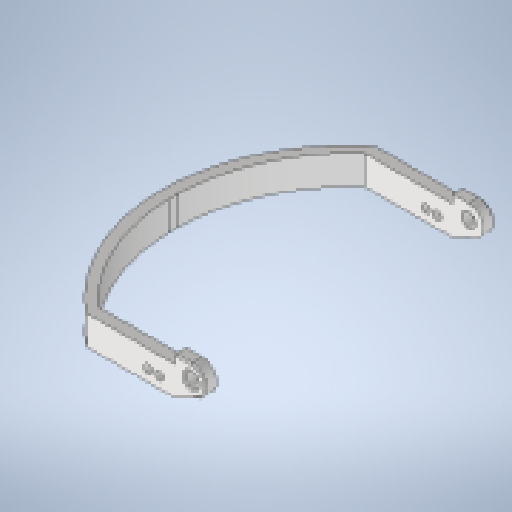
# Autodesk Inventor part: Gripper_v1
Saved by Autodesk Inventor 2025.1 (Build 291241000, 241)
## iProperties
Created: 2026-05-06
Part Number: Gripper_v1
Material: Generic
Document SubType Name: Modeling
Designer: User
Density: 1 g/cm^3
Appearance: Default
Author: User
## iProperties of the stored document Gripper_v1_3DPrint.ipt
Created: 2026-05-06
Part Number: Gripper_v1_3DPrint
Material: Generic
Document SubType Name: Modeling
Designer: User
Density: 1 g/cm^3
Appearance: Default
Author: User
Autodesk Inventor part; units mm, degrees
ref_plane "YZ Plane" through (0, 0, 0) normal (1, 0, 0) x (0, 1, 0)
ref_plane "XZ Plane" through (0, 0, 0) normal (0, 1, 0) x (-1, 0, 0)
ref_plane "XY Plane" through (0, 0, 0) normal (0, 0, 1) x (1, 0, 0)
sketch "Sketch1" plane through (0, 0, 0) normal (0, 0, 1) x (1, 0, 0)
  circle A0 centre (0, 0) radius 2.5 projected
  circle A1 centre (0, 0) radius 2.6
  circle A2 centre (0, 0) radius 5.1
  point P0 (0, 0)
  dimension "d0" = 0.1
  dimension "d1" = 2.5
  constraints: 2 centre point
  measures "d0" radial gap between concentric circles of A0 A1
  measures "d1" radial gap between concentric circles of A1 A2
ref_plane "Work Plane1" through (-3.6464, -27.211, -4) normal (0, 0, 1) x (1, 0, 0)
extrude "Extrusion1" add sketch "Sketch1" against normal up to surface (4 mm away) contours A2
chamfer "Chamfer1" distance 0.5 angle 45 1 edges at (-2.6, 0, -4)
sketch "Sketch2" plane through (0, 0, 0) normal (0, 0, 1) x (1, 0, 0)
  circle A0 centre (0, 0) radius 5.1 projected
  line L0 (-5.6464, 6) -> (-5.6464, -27.211) projected
  circle A1 centre (0, 0) radius 5.1 projected
  line L1 (0, -5.1) -> (-5.6464, -5.1)
  line L2 (0, 5.1) -> (-5.6464, 5.1)
  point P0 (0, 0)
  constraints: 4 end point, 3 tangent, 2 perpendicular, 2 point on circle, 2 point on line
extrude "Extrusion2" add sketch "Sketch2" against normal up to surface (4 mm away) contours A0 L1 L0 L2
sketch "Sketch5" plane through (-5.6464, -5.1, 0) normal (-1, 0, 0) x (0, 0, 1)
  line L0 (-4, 0) -> (-4, 10.2) projected
  line L1 (0, 0) -> (-4, 0) projected
  line L2 (0, 10.2) -> (0, 0) projected
  line L3 (0, 10.2) -> (-4, 10.2) projected
  line L4 (0, 0) -> (0, -3)
  line L5 (0, -3) -> (-4, -3)
  line L6 (-4, 10.2) -> (-4, 7.2)
  line L7 (-4, 7.2) -> (0, 7.2)
  line L8 (0, 7.2) -> (0, -3)
  line L9 (0, -3) -> (-4, -3)
  line L10 (-4, -3) -> (-4, 7.2)
  point P0 (0, 5.1)
  dimension "d14" = 3
  dimension "d15" = 3
  constraints: 14 end point, 2 parallel, 2 perpendicular, 1 horizontal, 1 point on line, 1 vertical
  measures "d14" distance of L1.start L4.end
  measures "d15" distance of L0.end L6.end
extrude "Extrusion5" add sketch "Sketch5" along normal blind 1 contours L0 L7 L2 L1 | L1 L4 L5 L10
sketch "Sketch6" plane through (0, 0, 0) normal (0, 0, 1) x (1, 0, 0)
  line L0 (-5.6464, -5.1) -> (0, -5.1) projected
  line L1 (-5.6464, 6) -> (-5.6464, -27.211) projected
  line L2 (-5.6464, -8.1) -> (-6.6464, -8.1) projected
  line L3 (-5.6464, -8.1) -> (0, -5.1)
  point P0 (0, 0)
  constraints: 2 end point
extrude "Extrusion6" add sketch "Sketch6" against normal up to surface (4 mm away)
ref_plane "Work Plane2" through (0, 0, 93.3284) normal (0, 0, -1) x (0, -1, 0)
sketch "Sketch7" plane through (0, 0, 93.3284) normal (0, 0, -1) x (0, -1, 0)
  arc A0 (-5.1, 0) -> (5.1, 0) centre (0, 0) ccw projected
  line L0 (-5.1, 0) -> (-5.1, 5.6464) projected
  line L1 (-5.1, 5.6464) -> (-2.1, 5.6464) projected
  line L2 (-2.1, 5.6464) -> (-2.1, 6.6464) projected
  line L3 (8.1, 6.6464) -> (-2.1, 6.6464) projected
  line L4 (8.1, 5.6464) -> (8.1, 6.6464) projected
  line L5 (8.1, 5.6464) -> (5.1, 0) projected
  circle A1 centre (0, 0) radius 2.6 projected
  point P0 (0, 0)
extrude "Extrusion7" add sketch "Sketch7" against normal blind 4
chamfer "Chamfer2" distance 0.5 angle 45 1 edges at (0, 2.6, 97.3284)
sketch "Sketch8" plane through (-6.6464, 2.1, 93.3284) normal (0, 1, 0) x (1, 0, 0)
  circle A0 centre (-3.5566, 46.3232) radius 35
  line L0 (1, 93.3284) -> (0, 93.3284) projected
  line L1 (1, 93.3284) -> (-8.6081, 93.3284)
  line L2 (0, 93.3284) -> (0, 97.3284) projected
  line L3 (1, 97.3284) -> (0, 97.3284) projected
  line L4 (0, 97.3284) -> (-3.5566, 97.3284)
  line L5 (0, 97.3284) -> (3.5566, 97.3284) construction
  line L6 (0, 0) -> (0, -4) projected
  line L7 (-3.5566, 93.3284) -> (-3.5566, 0)
  arc A1 (-3.5566, 93.3284) -> (-3.5566, 0) centre (-3.5566, 46.6642) ccw
  arc A2 (0, 97.2034) -> (-3.5566, -4) centre (-3.5566, 46.6642) ccw
  line L8 (0, -4) -> (-3.5566, -4)
  line L9 (0, -4) -> (3.5566, -4) construction
  line L10 (-3.5566, -4) -> (-3.5566, 0)
  line L11 (-3.5566, 0) -> (0, 0)
  line L12 (0, 93.3284) -> (-30, 93.3284)
  line L13 (0, 93.3284) -> (30, 93.3284) construction
  line L14 (0, 97.3284) -> (-30, 97.3284)
  line L15 (0, 97.3284) -> (30, 97.3284) construction
  line L16 (-30, 97.3284) -> (-30, 93.3284)
  line L17 (0, 0) -> (-30, 0)
  line L18 (0, 0) -> (30, 0) construction
  line L19 (0, -4) -> (-30, -4)
  line L20 (0, -4) -> (30, -4) construction
  line L21 (-30, -4) -> (-30, 0)
  line L22 (-30, 93.3284) -> (-30, 0)
  arc A3 (-30, 93.3284) -> (-30, 0) centre (13.7629, 46.6642) ccw
  arc A4 (-30, 97.3284) -> (-30, -4) centre (10.8784, 46.6642) ccw
  point P0 (6.6464, 93.3284)
  point P1 (-50.1868, 44.8848)
  point P2 (-50.1868, 48.4436)
  point P3 (-3.5566, -4)
  dimension "d25" = 180
  dimension "d26" = 180
  dimension "d29" = 30
  dimension "d30" = 180
  dimension "d31" = 30
  dimension "d32" = 180
  dimension "d33" = 30
  dimension "d34" = 180
  dimension "d35" = 30
  dimension "d36" = 180
  constraints: 38 end point, 10 horizontal, 9 point on circle, 7 collinear, 5 centre point, 2 perpendicular, 2 point on line, 1 coincident, 1 midpoint, 2 other
  measures "d25" angle of L4 L5
  measures "d26" angle of L8 L9
  measures "d29" distance of L0.end L12.end
  measures "d30" angle of L13 L12
  measures "d31" distance of L2.end L14.end
  measures "d32" angle of L14 L15
  measures "d33" distance of L6.start L17.end
  measures "d34" angle of L17 L18
  measures "d35" distance of L6.end L19.end
  measures "d36" angle of L19 L20
extrude "Extrusion8" add sketch "Sketch8" against normal up to surface (10.2 mm away) contours L1 L12 A2 L2 | L11 L6 L8 L10 | L10 A2 L17 | L19 L21 L17 A2 | A1 A3 A2 | A2 L4 L2 | L12 L16 L14 A2 | A4 A2 A3 L21 | A2 A4 L16 A3
sketch "Sketch9" plane through (0, 0, 0) normal (0, 0, 1) x (1, 0, 0)
  circle A0 centre (-11.0326, -4.1) radius 1.5 projected
  line L0 (-11.0326, -4.1) -> (-15.0326, -4.1)
  line L1 (-11.0326, -4.1) -> (-7.0326, -4.1) construction
  circle A1 centre (-15.0326, -4.1) radius 1.5
  point P0 (0, 0)
  dimension "d45" = 4
  dimension "d46" = 180
  dimension "d47" = 3
  constraints: 4 end point, 2 horizontal, 1 centre point, 1 coincident, 1 collinear
  measures "d45" distance of L0.start L0.end
  measures "d46" angle of L0 L1
  measures "d47" diameter of A1
extrude "Extrusion9" cut sketch "Sketch9" along normal through all both and the other way through all
chamfer "Chamfer3" distance 0.5 angle 45 2 edges at (5.1, 0, -4) (-2.8232, 5.1, -4)
chamfer "Chamfer4" distance 0.5 angle 45 2 edges at (5.1, 0, 97.3284) (-2.8232, 5.1, 97.3284)
sketch "Sketch10" plane through (0, 0, 97.3284) normal (0, 0, 1) x (1, 0, 0)
  line L0 (-36.6464, -8.1) -> (-5.6464, -8.1) projected
  circle A0 centre (-15.0326, -4.1) radius 1.5 projected
  line L1 (-15.0326, -4.1) -> (-15.0326, -8.1)
  line L2 (-15.0326, -4.1) -> (-15.0326, -14.1)
  circle A1 centre (-15.0326, -14.1) radius 1.5
  line L3 (-5.6464, -8.1) -> (1.2866, -4.4164) projected
  line L4 (-15.0326, -8.1) -> (-21.0326, -8.1)
  circle A2 centre (-15.0326, -14.1) radius 3
  line L5 (-21.0326, -8.1) -> (-21.0326, -12.1)
  line L6 (-21.0326, -8.1) -> (-17.0326, -8.1) construction
  line L7 (-16.0326, -17.1) -> (-15.0326, -17.1)
  line L8 (-5.6464, -8.1) -> (-12.7958, -16.0992)
  arc A3 (-21.0326, -12.1) -> (-16.0326, -17.1) centre (-16.0326, -12.1) ccw
  point P0 (0, 0)
  dimension "d48" = 10
  dimension "d49" = 3
  dimension "d50" = 6
  dimension "d51" = 6
  dimension "d52" = 90
  dimension "d53" = 5
  constraints: 14 end point, 4 point on circle, 4 tangent, 3 centre point, 3 point on line, 2 coincident, 2 perpendicular, 1 horizontal
  measures "d48" distance of L1.start L2.end
  measures "d49" diameter of A1
  measures "d50" distance of L1.end L4.end
  measures "d51" diameter of A2
  measures "d52" angle of L5 L6
  measures "d53" radius of A3
extrude "Extrusion10" add sketch "Sketch10" against normal up to surface (4 mm away) contours L0 L2 A2 L7 A3 L5 | L0 L8 A2 L2 | A2
chamfer "Chamfer5" distance 4 angle 45 1 edges at (-21.0326, -8.1, 95.3284)
sketch "Sketch11" plane through (0, 0, 0) normal (0, 0, 1) x (1, 0, 0)
  line L0 (-5.6464, -8.1) -> (-36.6464, -8.1) projected
  line L1 (-21.0326, -12.1) -> (-25.0326, -8.1) projected
  arc A0 (-21.0326, -12.1) -> (-16.0326, -17.1) centre (-16.0326, -12.1) ccw projected
  arc A1 (-15.0326, -17.1) -> (-12.7958, -16.0992) centre (-15.0326, -14.1) ccw projected
  circle A2 centre (-15.0326, -14.1) radius 1.5 projected
  line L2 (-12.7958, -16.0992) -> (-5.6464, -8.1) projected
  line L3 (-16.0326, -17.1) -> (-15.0326, -17.1) projected
  point P0 (0, 0)
extrude "Extrusion11" add sketch "Sketch11" against normal up to surface (4 mm away)
sketch "Sketch12" plane through (0, 0, 97.3284) normal (0, 0, 1) x (1, 0, 0)
  line L0 (-5.2661, -5.4078) -> (-11.5866, -16.1311) projected
  arc A0 (-18.4785, -12.0689) -> (-11.5866, -16.1311) centre (-15.0326, -14.1) ccw projected
  arc A1 (-21.0326, -12.1) -> (-16.0326, -17.1) centre (-16.0326, -12.1) ccw projected
  line L1 (-19.0326, -16.1) -> (-17.4326, -17.3)
  line L2 (-16.0326, -17.1) -> (-15.0326, -17.1) projected
  arc A2 (-15.0326, -17.1) -> (-12.7958, -16.0992) centre (-15.0326, -14.1) ccw projected
  line L3 (-12.7958, -16.0992) -> (-5.6464, -8.1) projected
  point P0 (0, 0)
  point P1 (-9.1897, -12.0645)
  constraints: 2 end point, 2 point on circle, 2 tangent
extrude "Extrusion12" add sketch "Sketch12" against normal up to surface (4 mm away)
sketch "Sketch13" plane through (-5.6464, 2.1, -4) normal (0, 0, -1) x (-1, 0, 0)
  circle A0 centre (9.3862, -16.2) radius 1.5 projected
  line L0 (-6.933, -6.5164) -> (0, -10.2) projected
  line L1 (0, -10.2) -> (7.1494, -18.1992) projected
  arc A1 (7.1494, -18.1992) -> (9.3862, -19.2) centre (9.3862, -16.2) ccw projected
  line L2 (9.3862, -19.2) -> (10.3862, -19.2) projected
  arc A2 (10.3862, -19.2) -> (15.3862, -14.2) centre (10.3862, -14.2) ccw projected
  line L3 (15.3862, -14.2) -> (19.3862, -10.2) projected
  line L4 (19.3862, -10.2) -> (31, -10.2) projected
  line L5 (31, 0) -> (31, -10.2) projected
  line L6 (0, 0) -> (31, 0) projected
  line L7 (0, 0) -> (0, 2.5) projected
  line L8 (-5.6464, 2.5) -> (0, 2.5) projected
  arc A3 (-5.6464, 2.5) -> (-6.933, -6.5164) centre (-5.6464, -2.1) ccw projected
  circle A4 centre (5.3862, -6.2) radius 1.5 projected
  circle A5 centre (9.3862, -6.2) radius 1.5 projected
  circle A6 centre (-5.6464, -2.1) radius 3.1 projected
  circle A7 centre (9.3862, -16.2) radius 1.5 projected
  circle A8 centre (3.0657, -5.4767) radius 1.5 projected
  line L9 (-0.9574, 22.62) -> (7.0426, 22.6266) projected
  line L10 (-0.9574, 22.62) -> (-0.9343, -5.48) projected
  arc A9 (-0.9343, -5.48) -> (-0.3803, -7.5078) centre (3.0657, -5.4767) ccw projected
  line L11 (-0.3803, -7.5078) -> (5.9402, -18.2311) projected
  arc A10 (5.9402, -18.2311) -> (12.8322, -14.1689) centre (9.3862, -16.2) ccw projected
  line L12 (12.8322, -14.1689) -> (7.0648, -4.384) projected
  line L13 (7.0648, -4.384) -> (7.0426, 22.6266) projected
  line L14 (13.3862, -18.2) -> (11.7862, -19.4) projected
  point P0 (-5.6464, -2.1)
  point P1 (3.5433, -14.1645)
extrude "Extrusion13" add sketch "Sketch13" against normal up to surface (4 mm away) contours L1 A1 L2 A2 A10 L11 | A10 A2 L14
sketch "Sketch14" plane through (-5.6464, 2.1, 0) normal (0, 1, 0) x (1, 0, 0)
  line L0 (12.1964, 1.0887) -> (49.0518, -35.7667) projected
  line L1 (34.6518, -71.5617) -> (12.1964, -94.0171) projected
  line L2 (34.3752, -71.8382) -> (-0.8463, -107.0598)
  line L3 (47.5716, -34.2865) -> (-11.9337, 25.2188)
  line L4 (5.6464, 4) -> (10.2464, 4) projected
  line L5 (10.7464, 3.5) -> (10.2464, 4) projected
  line L6 (10.7464, 0) -> (10.7464, 3.5) projected
  line L7 (10.7464, -96.8284) -> (10.2464, -97.3284) projected
  line L8 (10.7464, -93.3284) -> (10.7464, -96.8284) projected
  line L9 (10.2464, -97.3284) -> (5.6464, -97.3284) projected
  point P0 (5.6464, 0)
  point P1 (6.933, 4)
  point P2 (6.933, -97.3284)
  point P3 (9.2851, 4)
  point P4 (10.7464, 2.5387)
  point P5 (10.7464, -95.4671)
  point P6 (8.8851, -97.3284)
  constraints: 4 end point, 4 point on line
extrude "Extrusion14" cut sketch "Sketch14" along normal mid plane 15
body "Solid1"
